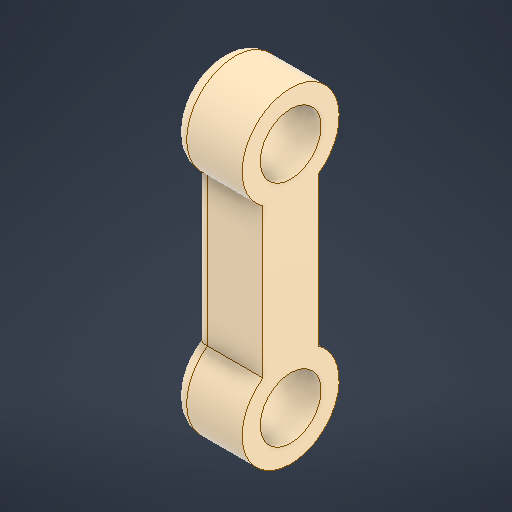
# Autodesk Inventor part: Barra_dedo
Saved by Autodesk Inventor 2027 (Build 310192060, 192F)
## iProperties
Created: 2026-06-13
Part Number: Barra_dedo
Material: Genérico
Document SubType Name: Modeling
Designer: angel
Density: 1 g/cm^3
Appearance: Suave - Color hueso
Author: angel
Autodesk Inventor part; units mm, degrees
ref_plane "YZ Plane" through (0, 0, 0) normal (1, 0, 0) x (0, 1, 0)
ref_plane "XZ Plane" through (0, 0, 0) normal (0, 1, 0) x (-1, 0, 0)
ref_plane "XY Plane" through (0, 0, 0) normal (0, 0, 1) x (1, 0, 0)
sketch "Boceto1" plane through (0, 0, 0) normal (1, 0, 0) x (0, 1, 0)
  circle A0 centre (0, 0) radius 2.2
  circle A1 centre (0, 0) radius 3.5
  line L0 (-3.5, 0) -> (16.5, 0)
  circle A2 centre (16.5, 0) radius 2.2
  circle A3 centre (16.5, 0) radius 3.5
  line L1 (2.8723, 2) -> (13.6277, 2)
  line L2 (2.8723, -2) -> (13.6277, -2)
  dimension "d0" = 4.4
  dimension "d1" = 7
  dimension "d2" = 20
  dimension "d3" = 4.4
  dimension "d4" = 7
  constraints: 6 end point, 5 point on circle, 4 centre point, 4 coincident, 2 horizontal, 1 parallel
  measures "d0" diameter of A0
  measures "d1" diameter of A1
  measures "d2" distance of L0.start L0.end
  measures "d3" diameter of A2
  measures "d4" diameter of A3
extrude "Extrusión1" add sketch "Boceto1" along normal blind 5 contours L0 A1 A0 | A0 L0 A1 | L0 A3 L2 A1 | A1 L1 A3 L0 | A3
fillet "Empalme2" radius 1 4 edges at (0, 8.25, -2) (0, 8.25, 2) (0, 20, 0) (0, -3.5, 0)
